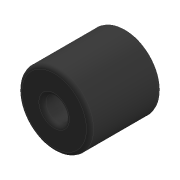
# Autodesk Inventor part: rubber
Saved by Autodesk Inventor 2020.3 (Build 243373000, 373)
## iProperties
Created: 2020-09-17
Part Number: rubber
Material: Rubber
Document SubType Name: Modeling
Designer: Svend
Density: 0.93 g/cm^3
Appearance: Rubber - Black
Author: Svend
Autodesk Inventor part; units mm, degrees
ref_plane "YZ Plane" through (0, 0, 0) normal (1, 0, 0) x (0, 1, 0)
ref_plane "XZ Plane" through (0, 0, 0) normal (0, 1, 0) x (-1, 0, 0)
ref_plane "XY Plane" through (0, 0, 0) normal (0, 0, 1) x (1, 0, 0)
sketch "Sketch1" plane through (0, 0, 0) normal (0, 0, 1) x (1, 0, 0)
  circle A0 centre (0, 0) radius 10
  circle A1 centre (0, 0) radius 3.25
  dimension "d0" = 20
  dimension "d1" = 6.5
  constraints: 2 centre point, 2 coincident
  measures "d0" diameter of A0
  measures "d1" diameter of A1
extrude "Extrusion1" add sketch "Sketch1" along normal mid plane 20
fillet "Fillet1" radius 1 4 edges at (-10, 0, 10) (-3.25, 0, 10) (-3.25, 0, -10) (-10, 0, -10)
body "Solid1"
